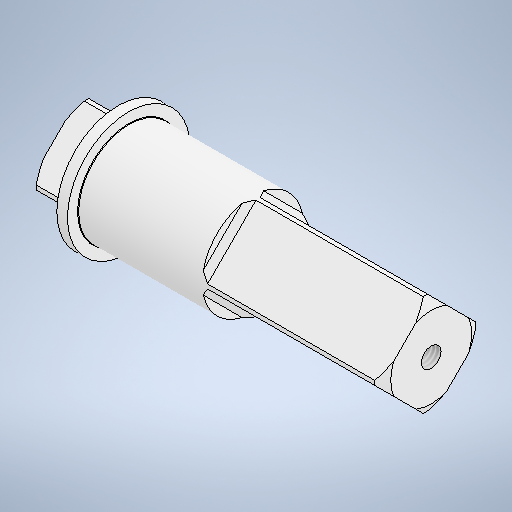
# Autodesk Inventor part: joint4_axis2
Saved by Autodesk Inventor 2025.3 (Build 293356030, 356C)
## iProperties
Created: 2025-10-28
Part Number: joint4_axis2
Material: PLA filament
Document SubType Name: Modeling
Designer: MSI
Density: 1.2 g/cm^3
Appearance: 일반
Mass: 17.1081 g
Surface Area: 50.7819 cm^2
Volume: 14.2568 cm^3
Author: MSI
Autodesk Inventor part; units mm, degrees
ref_plane "YZ Plane" through (0, 0, 0) normal (1, 0, 0) x (0, 1, 0)
ref_plane "XZ Plane" through (0, 0, 0) normal (0, 1, 0) x (-1, 0, 0)
ref_plane "XY Plane" through (0, 0, 0) normal (0, 0, 1) x (1, 0, 0)
sketch "스케치2" plane through (0, 0, 0) normal (0, 0, 1) x (1, 0, 0)
  line L0 (0, 0) -> (7, 0)
  line L1 (7, 0) -> (7, 9.5)
  line L2 (7, 9.5) -> (0, 9.5)
  line L3 (0, 9.5) -> (0, 0)
  line L4 (7, 0) -> (9, 0)
  line L5 (9, 0) -> (9, 11.5)
  line L6 (9, 11.5) -> (7, 11.5)
  line L7 (7, 11.5) -> (7, 0)
  line L8 (9, 0) -> (65.803, 0)
  line L9 (65.803, 0) -> (65.803, 9.5)
  line L10 (65.803, 9.5) -> (9, 9.5)
  line L11 (9, 9.5) -> (9, 0)
  point P0 (9, 9.5)
  point P1 (7, 9.5)
  dimension "d0" = 19
  dimension "d1" = 23
  dimension "d2" = 65.803
  dimension "d3" = 2
  dimension "d4" = 7
  constraints: 24 end point, 6 parallel, 3 horizontal, 3 perpendicular, 1 collinear
  measures "d0" diameter of L2 L0
  measures "d1" diameter of L6 L4
  measures "d2" distance between parallel lines of L9 L3
  measures "d3" distance of L5.end L6.end
  measures "d4" distance of L1.end L2.end
revolve "회전1" add sketch "스케치2" angle 360 about axis through (9, 0, 0) along (1, 0, 0)
chamfer "모따기1" distance 1.9 angle 30 1 edges at (0, -9.5, 0) measured on face at (0, -9, 0)
sketch "스케치3" plane through (0, 0, 0) normal (-1, 0, 0) x (0, 0, 1)
  line L0 (0, -9.8995) -> (9.8995, 0)
  line L1 (9.8995, 0) -> (0, 9.8995)
  line L2 (0, 9.8995) -> (-9.8995, 0)
  line L3 (-9.8995, 0) -> (0, -9.8995)
  line L4 (0, -9.8995) -> (0, 9.8995) construction
  line L5 (9.8995, 0) -> (-9.8995, 0) construction
  circle A0 centre (0, 0) radius 9.5 projected
  point P0 (0, 0)
  point P1 (-9.4912, -0.4083)
  point P2 (-9.4912, 0.4083)
  point P3 (-0.4083, 9.4912)
  point P4 (0.4083, 9.4912)
  point P5 (0.4083, -9.4912)
  point P6 (-0.4083, -9.4912)
  point P7 (9.4912, 0.4083)
  point P8 (9.4912, -0.4083)
  dimension "d9" = 14
  constraints: 12 end point, 2 midpoint, 2 parallel, 1 horizontal, 1 perpendicular, 1 vertical
  measures "d9" distance of L1.end L2.end
extrude "돌출1" cut sketch "스케치3" against normal up to surface (7 mm away) contours L3 A0 L0 | L0 A0 | A0 L3 | A0 L1 L0 | L3 L2 A0 | A0 L2 | L1 A0 | L2 L1 A0
fillet "모깎기1" radius 0.1 1 edges at (9, -9.5, 0)
chamfer "모따기2" distance 1.9 angle 30 1 edges at (65.803, -9.5, 0) measured on face at (65.803, -9, 0)
sketch "스케치4" plane through (65.803, 0, 0) normal (1, 0, 0) x (0, 0, -1)
  circle A0 centre (0, 0) radius 9.5 projected
  line L0 (0, -9.8995) -> (9.8995, 0)
  line L1 (9.8995, 0) -> (0, 9.8995)
  line L2 (0, 9.8995) -> (-9.8995, 0)
  line L3 (-9.8995, 0) -> (0, -9.8995)
  line L4 (0, -9.8995) -> (0, 9.8995) construction
  line L5 (9.8995, 0) -> (-9.8995, 0) construction
  point P0 (0, 0)
  point P1 (-0.4083, -9.4912)
  point P2 (-9.4912, -0.4083)
  point P3 (-9.4912, 0.4083)
  point P4 (-0.4083, 9.4912)
  point P5 (0.4083, 9.4912)
  point P6 (9.4912, 0.4083)
  point P7 (0.4083, -9.4912)
  point P8 (9.4912, -0.4083)
  dimension "d16" = 14
  constraints: 12 end point, 2 midpoint, 2 parallel, 1 horizontal, 1 perpendicular, 1 vertical
  measures "d16" distance of L1.end L2.end
extrude "돌출2" cut sketch "스케치4" against normal blind 33.5 contours A0 L1 L0 | L1 A0 | A0 L0 | A0 L2 L1 | L0 L3 A0 | L2 A0 | A0 L3 | A0 L3 L2
sketch "스케치5" plane through (0, 0, 0) normal (-1, 0, 0) x (0, 0, 1)
  circle A0 centre (0, 0) radius 11.5 projected
  point P0 (0, 0)
  point P1 (0, 0)
  constraints: 1 coincident
hole "구멍1" at (0, 0, 0) direction (1, 0, 0) diameter 9 depth 16
ref_plane "작업 평면1" through (16, 0, 0) normal (-1, 0, 0) x (0, 0, 1)
sketch "스케치6" plane through (16, 0, 0) normal (-1, 0, 0) x (0, 0, 1)
  line L0 (-2.8284, 3.5) -> (2.8284, 3.5)
  circle A0 centre (0, 0) radius 4.5 projected
  point P0 (0, 0)
  dimension "d26" = 3.5
  constraints: 2 end point, 2 point on circle, 1 horizontal
  measures "d26" distance from line of point (0, 0) L0
extrude "돌출3" add sketch "스케치6" along normal blind 9 contours A0 L0 picked at (0.2862, 4.0153)
chamfer "모따기3" distance 1 angle 45 1 edges at (0, 0, -4.5)
chamfer "모따기4" distance 1 angle 45 4 edges at (32.303, -4.9497, 4.9497) (32.303, -4.9497, -4.9497) (32.303, 4.9497, 4.9497) (32.303, 4.9497, -4.9497)
sketch "스케치8" plane through (65.803, 0, 0) normal (1, 0, 0) x (0, 0, -1)
  circle A0 centre (0, 0) radius 11.5 projected
  point P0 (0, 0)
  constraints: 1 coincident
hole "구멍3" at (65.803, 0, 0) direction (-1, 0, 0) diameter 3.6881 depth 13 tip angle 118 thread size "M4.5x0.75" class "6H" standard "ISO Metric profile"
equation "\"d0\" = joint4_axis2_d"
equation "\"d2\" = joint4_axis2_L + d4"
equation "\"d6\" = 0.1 * joint4_axis2_d"
equation "\"d13\" = 0.1 * joint4_axis2_d"
equation "\"joint4_belt_centor\" = 157.367"
equation "\"joint4_axis2_L\" = 58.803"
equation "\"joint4_axis2_b1\" = 35"
equation "\"joint4_axis2_d\" = 19"
equation "\"joint4_miter_m\" = 2"
equation "\"joint4_miter_a\" = 20deg"
equation "\"joint4_miter_z\" = 79"
equation "\"joint4_miter_b\" = 6.90139"
equation "\"joint4_axis3_L\" = 23.5"
equation "\"joint3_belt_centor\" = 157.367"
equation "\"joint3_axis2_L\" = 16"
equation "\"joint3_axis2_d\" = 19"
equation "\"joint3_planetary_m\" = 1.5"
equation "\"joint3_planetary_a\" = 20deg"
equation "\"joint3_planetary_np\" = 4"
equation "\"joint3_sun_z\" = 18"
equation "\"joint3_sun_b\" = 17"
equation "\"joint3_planet_z\" = 36"
equation "\"joint3_planet_b\" = 17"
equation "\"joint3_ring_b\" = 9"
equation "\"joint3_axis3_d\" = 29"
equation "\"joint3_miter_m\" = 5.5"
equation "\"joint3_miter_a\" = 20deg"
equation "\"joint3_miter_z\" = 28"
equation "\"joint3_miter_b\" = 13.65957"
equation "\"joint3_axis4_L\" = 23.5"
